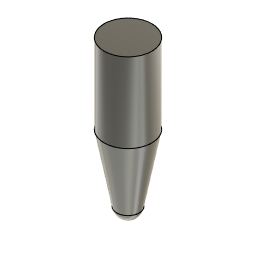
SimonStrachan_Aluminiumblock_v1 (Autodesk Fusion 360 archive; units mm, degrees)
design "eppendorf_cutout"
Autodesk Fusion 360 part; units mm, degrees
sketch "Sketch1" plane through (0, 0, 0) normal (1, 0, 0) x (0, 1, 0)
  line L0 (0, 0) -> (0, 37.5)
  line L1 (0, 37.5) -> (5.7, 37.5)
  line L2 (5.7, 37.5) -> (5.7, 18.5)
  line L3 (0, 0) -> (0, 2.5)
  line L4 (2.7, 2.5) -> (5.7, 18.5)
  arc A0 (0, 0) -> (2.7, 2.5) centre (-0.3342, 3.0689) ccw
  dimension "d1" = 37.5
  dimension "d2" = 5.7
  dimension "d3" = 19
  dimension "d4" = 2.5
  dimension "d5" = 2.7
  constraint coincident L0.start L3.start
  constraint vertical L0
  constraint perpendicular L0 L1
  constraint vertical L2
  constraint parallel L0 L3
  constraint tangent L4 A0
  measures "d1" distance of L0.start L0.end
  measures "d2" distance of L0.end L1.end
  measures "d3" distance of L1.end L2.end
  measures "d4" distance of L0.start L3.end
  measures "d5" distance of L3.end L4.start
revolve "Revolve1" add sketch "Sketch1" angle 360 about axis through (0, 0, 0) along (0, 0, 1)
